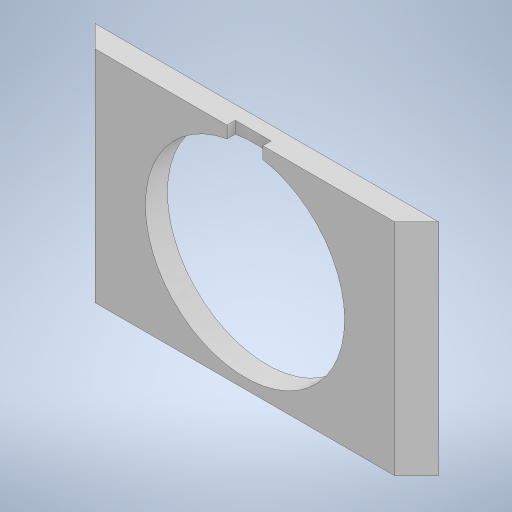
# Autodesk Inventor part: org_case_psu_connector
Saved by Autodesk Inventor 2024 (Build 280153000, 153)
## iProperties
Created: 2023-07-13
Part Number: org_case_psu_connector
Material: Generic
Document SubType Name: Modeling
Designer: jconvertino
Density: 1 g/cm^3
Appearance: Default
Author: jconvertino
Autodesk Inventor part; units mm, degrees
ref_plane "YZ Plane" through (0, 0, 0) normal (1, 0, 0) x (0, 1, 0)
ref_plane "XZ Plane" through (0, 0, 0) normal (0, 1, 0) x (-1, 0, 0)
ref_plane "XY Plane" through (0, 0, 0) normal (0, 0, 1) x (1, 0, 0)
sketch "Sketch1" plane through (0, 0, 0) normal (0, 0, 1) x (1, 0, 0)
  line L0 (0, 0) -> (31.75, 0)
  line L1 (31.75, 0) -> (31.75, 20.32)
  line L2 (31.75, 20.32) -> (0, 20.32)
  line L3 (0, 20.32) -> (0, 0)
  circle A0 centre (15.875, 10.16) radius 9.2075
  dimension "d0" = 20.32
  dimension "d1" = 31.75
  dimension "d2" = 15.875
  dimension "d3" = 15.875
  dimension "d4" = 10.16
  dimension "d5" = 10.16
  dimension "d6" = 18.415
  constraints: 8 end point, 2 parallel, 1 centre point, 1 horizontal, 1 perpendicular
  measures "d0" distance of L2.end L0.start
  measures "d1" distance of L0.start L0.end
  measures "d2" distance from line of L3 A0.centre
  measures "d3" distance from line of L1 A0.centre
  measures "d4" distance from line of L2 A0.centre
  measures "d5" distance from line of L0 A0.centre
  measures "d6" diameter of A0
extrude "Extrusion1" add sketch "Sketch1" along normal blind 2.032
chamfer "Chamfer2" distance 2.032 angle 45 2 edges at (0, 10.16, 2.032) (31.75, 10.16, 2.032)
sketch "Sketch2" plane through (0, 0, 2.032) normal (0, 0, 1) x (1, 0, 0)
  line L0 (14.224, 21.0828) -> (17.526, 21.0828)
  line L1 (17.526, 21.0828) -> (17.526, 18.4625)
  line L2 (17.526, 18.4625) -> (14.224, 18.4625)
  line L3 (14.224, 18.4625) -> (14.224, 21.0828)
  line L4 (2.032, 0) -> (2.032, 20.32) projected
  line L5 (29.718, 20.32) -> (29.718, 0) projected
  point P0 (0, 0)
  point P1 (14.224, 19.7726)
  dimension "d15" = 12.192
  dimension "d16" = 12.192
  constraints: 8 end point, 2 parallel, 1 horizontal, 1 midpoint, 1 perpendicular
  measures "d15" distance from line of point (14.224, 19.773) L4
  measures "d16" distance between parallel lines of L5 L1
extrude "Extrusion2" cut sketch "Sketch2" against normal blind 0.762
body "Solid1"
